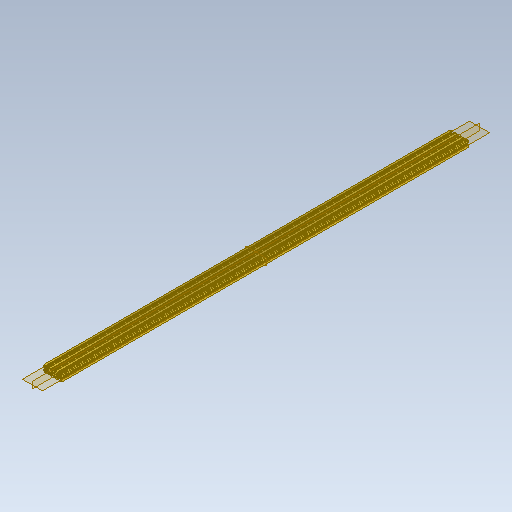
# Autodesk Inventor part: Perfil 30×60 6 rasgos_AST03006006
Saved by Autodesk Inventor 2025.2 (Build 292293000, 293)
## iProperties
Created: 2025-04-06
Part Number: Perfil 30×60 6 rasgos_AST03006006
Material: Ouro
Document SubType Name: Modeling
Designer: Gustavo Sousa
Density: 19.3 g/cm^3
Appearance: Metal quente 2400F
Author: Gustavo Sousa
Autodesk Inventor part; units mm, degrees
sketch "Esboço1" plane through (0, 0, 0) normal (0, 0, 1) x (1, 0, 0)
  line L0 (-45, 15) -> (45, 15) construction
  circle A0 centre (-30, 0) radius 5 construction
  line L1 (-30, 0) -> (-15, 15) construction
  line L2 (-37, 7) -> (-23, 7) construction
  line L3 (-34.1, 15) -> (-25.9, 15) construction
  line L4 (-45, 15) -> (-30, 15) construction
  line L5 (-37, 7) -> (-37, 0) construction
  line L6 (-45, 15) -> (-45, -15) construction
  line L7 (-34.1, 15) -> (-34.6, 15) construction
  line L8 (-34.6, 15) -> (-34.6, 14.5)
  line L9 (-34.6, 14.5) -> (-34.1, 14.5)
  line L10 (-34.1, 14.5) -> (-34.1, 15) construction
  line L11 (-34.1, 15) -> (-34.1, 12.8) construction
  line L12 (-34.1, 12.8) -> (-38.15, 12.8) construction
  line L13 (-34.1, 14.5) -> (-34.1, 12.8)
  line L14 (-37, 7) -> (-30, 0) construction
  line L15 (-37, 7) -> (-45, 15) construction
  arc A1 (-44.5, 15) -> (-45, 14.5) centre (-44.5, 14.5) ccw construction
  arc A2 (-44.5, 15) -> (-44.8536, 14.8536) centre (-44.5, 14.5) ccw
  line L16 (-44.5, 15) -> (-34.6, 15)
  line L17 (-38.15, 9.7056) -> (-35.4444, 7) construction
  line L18 (-38.15, 12.8) -> (-38.15, 9.7056) construction
  line L19 (-35.4444, 7) -> (-30, 7) construction
  circle A3 centre (-41.5, 11.5) radius 2.25 construction
  line L20 (-25.9, 15) -> (-25.4, 15) construction
  line L21 (-25.4, 15) -> (-25.4, 14.5)
  line L22 (-25.4, 14.5) -> (-25.9, 14.5)
  line L23 (-25.9, 14.5) -> (-25.9, 15) construction
  line L24 (-25.9, 15) -> (-25.9, 12.8) construction
  line L25 (-25.9, 12.8) -> (-21.85, 12.8) construction
  line L26 (-25.9, 14.5) -> (-25.9, 12.8)
  line L27 (-24.5556, 7) -> (-21.85, 9.7056) construction
  line L28 (-21.85, 12.8) -> (-21.85, 9.7056) construction
  line L29 (-24.5556, 7) -> (-30, 7) construction
  line L30 (-23, 7) -> (-23, 0) construction
  line L31 (-37, 0) -> (-35, 0)
  line L32 (-25, 0) -> (-23, 0)
  line L33 (-19.65, 8.7944) -> (-23, 5.4444) construction
  arc A4 (-30, 5) -> (-35, 0) centre (-30, 0) ccw construction
  arc A5 (-25, 0) -> (-30, 5) centre (-30, 0) ccw
  line L34 (-19.65, 12.8) -> (-15, 12.8) construction
  line L35 (-19.65, 12.8) -> (-19.65, 8.7944) construction
  line L36 (-23, 5.4444) -> (-23, 0) construction
  arc A6 (-39.909, 9.909) -> (-43.091, 13.091) centre (-41.5, 11.5) ccw
  arc A7 (-30, 5) -> (-33.5355, 3.5355) centre (-30, 0) ccw
  line L37 (-44.8536, 14.8536) -> (-33.5355, 3.5355)
  line L38 (-30, 5) -> (-30, 7)
  line L39 (-25, 0) -> (-23, 0)
  arc A8 (-35.5908, 7.1464) -> (-35.2373, 7) centre (-35.2373, 7.5) ccw
  arc A9 (-38.15, 9.9127) -> (-38.0036, 9.5592) centre (-37.65, 9.9127) ccw
  arc A10 (-37.65, 12.8) -> (-38.15, 12.3) centre (-37.65, 12.3) ccw
  line L40 (-37.65, 12.8) -> (-34.1, 12.8)
  line L41 (-38.15, 12.3) -> (-38.15, 9.9127)
  line L42 (-38.0036, 9.5592) -> (-35.5908, 7.1464)
  line L43 (-35.2373, 7) -> (-30, 7)
  arc A11 (-21.85, 12.3) -> (-22.35, 12.8) centre (-22.35, 12.3) ccw
  arc A12 (-21.9964, 9.5592) -> (-21.85, 9.9127) centre (-22.35, 9.9127) ccw
  arc A13 (-24.7627, 7) -> (-24.4092, 7.1464) centre (-24.7627, 7.5) ccw
  line L44 (-25.9, 12.8) -> (-22.35, 12.8)
  line L45 (-21.85, 12.3) -> (-21.85, 9.9127)
  line L46 (-21.9964, 9.5592) -> (-24.4092, 7.1464)
  line L47 (-24.7627, 7) -> (-30, 7)
  arc A14 (-22.8536, 5.5908) -> (-23, 5.2373) centre (-22.5, 5.2373) ccw
  arc A15 (-19.7964, 8.6479) -> (-19.65, 9.0015) centre (-20.15, 9.0015) ccw
  arc A16 (-19.15, 12.8) -> (-19.65, 12.3) centre (-19.15, 12.3) ccw
  line L48 (-23, 5.2373) -> (-23, 0)
  line L49 (-22.8536, 5.5908) -> (-19.7964, 8.6479)
  line L50 (-19.65, 9.0015) -> (-19.65, 12.3)
  line L51 (-19.15, 12.8) -> (-15, 12.8)
  line L52 (-30, 15) -> (-15, 15) construction
  line L53 (-25.4, 15) -> (-15, 15)
  line L54 (-15, 15) -> (-15, 12.8)
  circle A17 centre (-33.5355, 3.5355) radius 1.1
  circle A18 centre (-26.4645, 3.5355) radius 1.1
  point P0 (0, 0)
  point P1 (-45, 0)
  point P2 (-25.9, 13.9)
  point P3 (-27.3231, 4.2231)
  point P4 (-25.7769, 2.6769)
  point P5 (-34.3134, 4.3134)
  point P6 (-32.6769, 4.2231)
  dimension "d0" = 15
  dimension "d1" = 90
  dimension "d4" = 10
  dimension "d6" = 8.2
  dimension "d7" = 15
  dimension "quadrado" = 0.5
  dimension "espessura" = 2.2
  dimension "d11" = 0.5
  dimension "d12" = 1.1
  dimension "d13" = 8
  dimension "d14" = 11.5
  dimension "d15" = 4.5
  dimension "d16" = 1.1
  dimension "d17" = 1.1
  dimension "d18" = 2
  dimension "d19" = 1.1
  dimension "d20" = 2.2
  dimension "d25" = 30
  dimension "d30" = 2.2
  dimension "d33" = 90
  constraints: 110 end point, 37 point on circle, 29 point on line, 24 tangent, 19 centre point, 14 collinear, 12 equal radius, 11 horizontal, 10 vertical, 7 parallel, 6 equal length, 6 perpendicular, 5 coincident, 5 horizontal alignment, 4 midpoint, 3 vertical alignment, 3 other
  measures "d0" distance from line of point (0, 0) L0
  measures "d1" distance of L0.start L0.end
  measures "d4" diameter of A0
  measures "d6" distance of L3.start L3.end
  measures "d7" distance of L0.start L4.end
  measures "quadrado" distance of L9.end L3.start
  measures "espessura" distance between parallel lines of L4 L12
  measures "d11" radius of A1
  measures "d12" distance between parallel lines of L15 L17
  measures "d13" distance of L4.end L19.end
  measures "d14" horizontal distance of L1.start A3.centre
  measures "d15" diameter of A3
  measures "d16" distance edge to line of A3 L18
  measures "d17" distance between parallel lines of L1 L27
  measures "d18" distance edge to line of A0 L5
  measures "d19" distance between parallel lines of L1 L33
  measures "d20" distance of L25.end L34.start
  measures "d25" distance of point (0, 0) L1.start
  measures "d30" diameter of A17
extrude "Extrusão4" add sketch "Esboço1" along normal mid plane 2000 contours L38 L47 A13 L46 A12 L45 A11 L44 L26 L22 L21 L53 L54 L51 A16 L50 A15 L49 A14 L48 L32 A5 A18
mirror "Espelhar5" about plane through (-15, 12.8, 0) normal (1, 0, 0) of "Extrusão4"
mirror "Espelhar6" about plane through (0, 0, 0) normal (0, 1, 0) of "Extrusão4", "Espelhar5"
mirror "Espelhar7" about plane through (0, 0, 0) normal (1, 0, 0) of "Extrusão4", "Espelhar5", "Espelhar6"
extrude "Extrusão3" add sketch "Esboço1" along normal mid plane 2000 contours L8 L9 L13 L40 A10 L41 A9 L42 A8 L43 L38 A7 A17 L37 A6 A2 L16
mirror "Espelhar8" about plane through (-44.8536, 14.8536, 0) normal (-0.7071068, -0.7071068, 0) of "Extrusão3"
mirror "Espelhar9" about plane through (0, 0, 0) normal (0, 1, 0) of "Extrusão3", "Espelhar8"
mirror "Espelhar10" about plane through (0, 0, 0) normal (1, 0, 0) of "Extrusão3", "Espelhar8", "Espelhar9"
equation "\"d12\" = 0.5 * espessura"
equation "\"d16\" = 0.5 * espessura"
equation "\"d17\" = 0.5 * espessura"
equation "\"d19\" = 0.5 * espessura"
